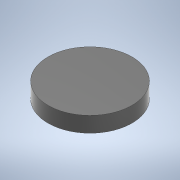
# Autodesk Inventor part: lidar
Saved by Autodesk Inventor 2022 (Build 260153000, 153)
## iProperties
Created: 2025-05-06
Part Number: lidar
Material: Ogólny
Document SubType Name: Modeling
Designer: Olga Kowalczyk IB 240875
Density: 1 g/cm^3
Appearance: Domyślna
Author: Olga Kowalczyk IB 240875
Autodesk Inventor part; units mm, degrees
ref_plane "YZ Plane" through (0, 0, 0) normal (1, 0, 0) x (0, 1, 0)
ref_plane "XZ Plane" through (0, 0, 0) normal (0, 1, 0) x (-1, 0, 0)
ref_plane "XY Plane" through (0, 0, 0) normal (0, 0, 1) x (1, 0, 0)
sketch "Szkic1" plane through (0, 0, 0) normal (0, 1, 0) x (-1, 0, 0)
  circle A0 centre (0, 0) radius 29.9
  arc A1 (42.6967, -16.4766) -> (42.6967, 16.4766) centre (36.8, 0) ccw
  arc A2 (-39.1229, 3.647) -> (-39.1229, -3.647) centre (-38.25, 0) ccw
  line L0 (42.6967, 16.4766) -> (10.075, 28.1515)
  line L1 (42.6967, -16.4766) -> (10.075, -28.1515)
  line L2 (-39.1229, 3.647) -> (-29.2918, 6)
  line L3 (-39.1229, -3.647) -> (-29.2918, -6)
  point P0 (54.3, 0)
  point P1 (29.9, 0)
  point P2 (-42, 0)
  dimension "d0" = 59.8
  dimension "d1" = 0
  dimension "d2" = 24.4
  dimension "d3" = 35
  dimension "d4" = 7.5
  dimension "d5" = 96.3
  dimension "d6" = 6
  dimension "d7" = 6
  constraints: 11 point on circle, 8 end point, 6 tangent, 4 horizontal alignment, 3 centre point, 1 coincident
  measures "d0" diameter of A0
  measures "d1" vertical distance of point (0, 0) A0.start
  measures "d2" distance of A0.start point (54.3, 0)
  measures "d3" diameter of A1
  measures "d4" diameter of A2
  measures "d5" distance of point (54.3, 0) point (-42, 0)
  measures "d6" vertical distance of A2.centre L2.end
  measures "d7" vertical distance of L3.end A2.centre
extrude "Wyciągnięcie proste2" add sketch "Szkic1" along normal blind 11 contours A0
